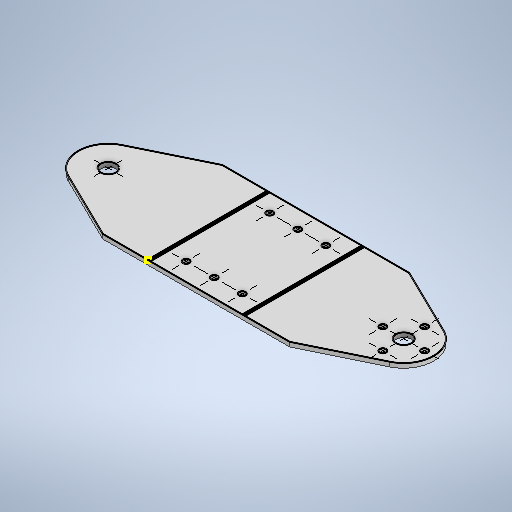
# Autodesk Inventor part: CAM_axis_6_bottom_frame(top)
Saved by Autodesk Inventor 2025.2 (Build 292293000, 293)
## iProperties
Created: 2025-08-09
Part Number: CAM_axis_6_bottom_frame(top)
Material: Generic
Document SubType Name: Modeling
Designer: User
Density: 1 g/cm^3
Appearance: Default
Author: User
Autodesk Inventor part; units mm, degrees
ref_plane "YZ Plane" through (0, 0, 0) normal (1, 0, 0) x (0, 1, 0)
ref_plane "XZ Plane" through (0, 0, 0) normal (0, 1, 0) x (-1, 0, 0)
ref_plane "XY Plane" through (0, 0, 0) normal (0, 0, 1) x (1, 0, 0)
sketch "Sketch1" plane through (0, 0, 0) normal (0, 1, 0) x (-1, 0, 0)
  line L0 (-32.1589, 0) -> (-32.1589, -40)
  line L1 (-0.4496, -40) -> (-0.4496, 0)
  circle A0 centre (-72.7986, -20) radius 1.05
  circle A1 centre (-65.7986, -13) radius 1.05
  circle A2 centre (-65.7986, -27) radius 1.05
  circle A3 centre (-58.7986, -20) radius 1.05
  circle A4 centre (-25.7093, -6) radius 1.05
  circle A5 centre (-25.7093, -34) radius 1.05
  circle A6 centre (-16.3043, -6) radius 1.05
  circle A7 centre (-16.3043, -34) radius 1.05
  circle A8 centre (-6.8993, -6) radius 1.05
  circle A9 centre (-6.8993, -34) radius 1.05
  circle A10 centre (-65.7986, -20) radius 2.6
  circle A11 centre (33.19, -20) radius 2.55
  line L2 (37.5744, -11.0124) -> (15, 0)
  arc A12 (37.5744, -28.9876) -> (37.5744, -11.0124) centre (33.19, -20) ccw
  line L3 (15, -40) -> (37.5744, -28.9876)
  line L4 (-47.6086, 0) -> (-70.183, -11.0124)
  arc A13 (-70.183, -11.0124) -> (-70.183, -28.9876) centre (-65.7986, -20) ccw
  line L5 (-70.183, -28.9876) -> (-47.6086, -40)
  line L6 (-47.6086, 0) -> (15, 0)
  line L7 (15, -40) -> (-47.6086, -40)
  line L8 (-32.6086, -40) -> (-32.6086, 0)
  line L9 (-31.7093, 0) -> (-31.7093, -40)
  line L10 (-0.8993, -40) -> (-0.8993, 0)
  line L11 (0, 0) -> (0, -40)
  constraints: 24 end point, 14 centre point, 12 point on line, 10 equal radius, 7 parallel, 6 vertical, 4 point on circle, 4 tangent, 2 horizontal, 2 perpendicular, 51 other
extrude "Extrusion1" add sketch "Sketch1" against normal blind 1.5
body "Solid1"
